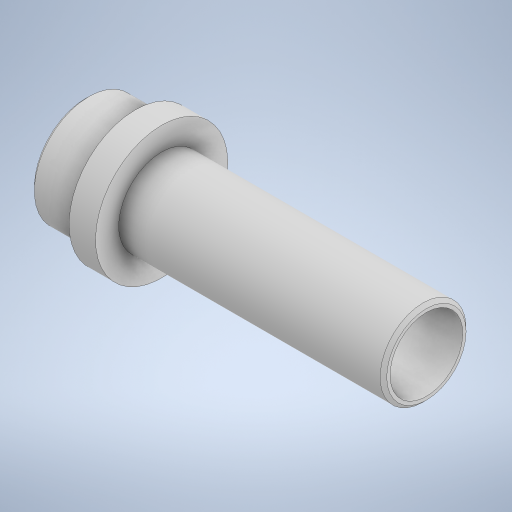
# Autodesk Inventor part: Bucha do Ferramental
Saved by Autodesk Inventor 2023 (Build 270158000, 158)
## iProperties
Created: 2022-04-25
Part Number: Bucha do Ferramental
Material: Generic
Document SubType Name: Modeling
Designer: coqui
Density: 1 g/cm^3
Appearance: Default
Author: coqui
Autodesk Inventor part; units mm, degrees
ref_plane "YZ Plane" through (0, 0, 0) normal (1, 0, 0) x (0, 1, 0)
ref_plane "XZ Plane" through (0, 0, 0) normal (0, 1, 0) x (-1, 0, 0)
ref_plane "XY Plane" through (0, 0, 0) normal (0, 0, 1) x (1, 0, 0)
sketch "Sketch1" plane through (0, 0, 0) normal (0, 0, 1) x (1, 0, 0)
  line L0 (-103, 11) -> (0, 11)
  line L1 (0, 11) -> (0, 12)
  line L2 (-1, 13) -> (-80, 13)
  line L3 (-80, 13) -> (-80, 20)
  line L4 (-80, 20) -> (-88, 20)
  line L5 (-103, 13) -> (-103, 11)
  line L6 (-103, 13) -> (-103, 15.5)
  line L7 (-102, 16.5) -> (-88, 16.5)
  line L8 (-88, 20) -> (-88, 16.5)
  line L9 (0, 12) -> (-1, 13)
  line L10 (-102, 16.5) -> (-103, 15.5)
  line L11 (-118.5, 0) -> (44.527, 0) construction
  point P0 (0, 0)
  point P1 (0, 13)
  point P2 (-84, 20)
  point P3 (-103, 16.5)
  dimension "d0" = 103
  dimension "d1" = 11
  dimension "d2" = 0
  dimension "d4" = 8
  dimension "d5" = 80
  dimension "d7" = 13
  dimension "d11" = 15
  dimension "d12" = 16.5
  dimension "d13" = 20
  dimension "d14" = 1
  dimension "d15" = 1
  dimension "d16" = 1
  dimension "d17" = 1
  constraints: 24 end point, 5 point on line, 3 perpendicular, 3 vertical, 2 horizontal, 1 midpoint
  measures "d0" distance of L0.start L0.end
  measures "d1" distance of point (0, 0) L0.end
  measures "d2" horizontal distance of point (0, 0) L0.end
  measures "d4" distance of L3.end L4.end
  measures "d5" distance of point (0, 13) L2.end
  measures "d7" distance of point (0, 0) point (0, 13)
  measures "d11" distance of point (-103, 16.5) L7.end
  measures "d12" distance from line of point (0, 0) L7
  measures "d13" vertical distance of point (0, 0) point (-84, 20)
  measures "d14" distance of L1.end point (0, 13)
  measures "d15" distance of L2.start point (0, 13)
  measures "d16" distance of L7.start point (-103, 16.5)
  measures "d17" distance of L6.end point (-103, 16.5)
revolve "Revolution1" add sketch "Sketch1" angle 360 about axis through (-118.5, 0, 0) along (1, 0, 0)
equation "\"d15\" = d14"
equation "\"d17\" = d16"
body "Solid1"
